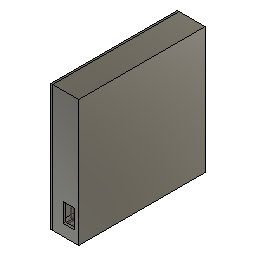
wifi-neopixel v1 (Autodesk Fusion 360 design; units mm, degrees)
Autodesk Fusion 360 part; units mm, degrees
(part 1 of 2)
sketch "Schizzo1" plane through (0, 0, 0) normal (1, 0, 0) x (0, 1, 0) in component "elettronica"
  line L0 (0, 0) -> (80, 0)
  line L1 (80, 0) -> (80, 80)
  line L2 (80, 80) -> (0, 80)
  line L3 (0, 80) -> (0, 0)
  line L4 (2, 77.5) -> (7, 77.5)
  line L5 (7, 77.5) -> (7, 72.5)
  line L6 (7, 72.5) -> (2, 72.5)
  line L7 (2, 72.5) -> (2, 77.5)
  line L8 (17, 72.5) -> (12, 72.5)
  line L9 (17, 77.5) -> (17, 72.5)
  line L10 (12, 77.5) -> (17, 77.5)
  line L11 (12, 72.5) -> (12, 77.5)
  line L12 (27, 72.5) -> (22, 72.5)
  line L13 (27, 77.5) -> (27, 72.5)
  line L14 (22, 77.5) -> (27, 77.5)
  line L15 (22, 72.5) -> (22, 77.5)
  line L16 (37, 72.5) -> (32, 72.5)
  line L17 (37, 77.5) -> (37, 72.5)
  line L18 (32, 77.5) -> (37, 77.5)
  line L19 (32, 72.5) -> (32, 77.5)
  line L20 (47, 72.5) -> (42, 72.5)
  line L21 (47, 77.5) -> (47, 72.5)
  line L22 (42, 77.5) -> (47, 77.5)
  line L23 (42, 72.5) -> (42, 77.5)
  line L24 (57, 72.5) -> (52, 72.5)
  line L25 (57, 77.5) -> (57, 72.5)
  line L26 (52, 77.5) -> (57, 77.5)
  line L27 (52, 72.5) -> (52, 77.5)
  line L28 (67, 72.5) -> (62, 72.5)
  line L29 (67, 77.5) -> (67, 72.5)
  line L30 (62, 77.5) -> (67, 77.5)
  line L31 (62, 72.5) -> (62, 77.5)
  line L32 (77, 72.5) -> (72, 72.5)
  line L33 (77, 77.5) -> (77, 72.5)
  line L34 (72, 77.5) -> (77, 77.5)
  line L35 (72, 72.5) -> (72, 77.5)
  line L36 (7, 62.5) -> (2, 62.5)
  line L37 (7, 67.5) -> (7, 62.5)
  line L38 (2, 67.5) -> (7, 67.5)
  line L39 (2, 62.5) -> (2, 67.5)
  line L40 (17, 62.5) -> (12, 62.5)
  line L41 (17, 67.5) -> (17, 62.5)
  line L42 (12, 67.5) -> (17, 67.5)
  line L43 (12, 62.5) -> (12, 67.5)
  line L44 (27, 62.5) -> (22, 62.5)
  line L45 (27, 67.5) -> (27, 62.5)
  line L46 (22, 67.5) -> (27, 67.5)
  line L47 (22, 62.5) -> (22, 67.5)
  line L48 (37, 62.5) -> (32, 62.5)
  line L49 (37, 67.5) -> (37, 62.5)
  line L50 (32, 67.5) -> (37, 67.5)
  line L51 (32, 62.5) -> (32, 67.5)
  line L52 (47, 62.5) -> (42, 62.5)
  line L53 (47, 67.5) -> (47, 62.5)
  line L54 (42, 67.5) -> (47, 67.5)
  line L55 (42, 62.5) -> (42, 67.5)
  line L56 (57, 62.5) -> (52, 62.5)
  line L57 (57, 67.5) -> (57, 62.5)
  line L58 (52, 67.5) -> (57, 67.5)
  line L59 (52, 62.5) -> (52, 67.5)
  line L60 (67, 62.5) -> (62, 62.5)
  line L61 (67, 67.5) -> (67, 62.5)
  line L62 (62, 67.5) -> (67, 67.5)
  line L63 (62, 62.5) -> (62, 67.5)
  line L64 (77, 62.5) -> (72, 62.5)
  line L65 (77, 67.5) -> (77, 62.5)
  line L66 (72, 67.5) -> (77, 67.5)
  line L67 (72, 62.5) -> (72, 67.5)
  line L68 (7, 52.5) -> (2, 52.5)
  line L69 (7, 57.5) -> (7, 52.5)
  line L70 (2, 57.5) -> (7, 57.5)
  line L71 (2, 52.5) -> (2, 57.5)
  line L72 (17, 52.5) -> (12, 52.5)
  line L73 (17, 57.5) -> (17, 52.5)
  line L74 (12, 57.5) -> (17, 57.5)
  line L75 (12, 52.5) -> (12, 57.5)
  line L76 (27, 52.5) -> (22, 52.5)
  line L77 (27, 57.5) -> (27, 52.5)
  line L78 (22, 57.5) -> (27, 57.5)
  line L79 (22, 52.5) -> (22, 57.5)
  line L80 (37, 52.5) -> (32, 52.5)
  line L81 (37, 57.5) -> (37, 52.5)
  line L82 (32, 57.5) -> (37, 57.5)
  line L83 (32, 52.5) -> (32, 57.5)
  line L84 (47, 52.5) -> (42, 52.5)
  line L85 (47, 57.5) -> (47, 52.5)
  line L86 (42, 57.5) -> (47, 57.5)
  line L87 (42, 52.5) -> (42, 57.5)
  line L88 (57, 52.5) -> (52, 52.5)
  line L89 (57, 57.5) -> (57, 52.5)
  line L90 (52, 57.5) -> (57, 57.5)
  line L91 (52, 52.5) -> (52, 57.5)
  line L92 (67, 52.5) -> (62, 52.5)
  line L93 (67, 57.5) -> (67, 52.5)
  line L94 (62, 57.5) -> (67, 57.5)
  line L95 (62, 52.5) -> (62, 57.5)
  line L96 (77, 52.5) -> (72, 52.5)
  line L97 (77, 57.5) -> (77, 52.5)
  line L98 (72, 57.5) -> (77, 57.5)
  line L99 (72, 52.5) -> (72, 57.5)
  line L100 (7, 42.5) -> (2, 42.5)
  line L101 (7, 47.5) -> (7, 42.5)
  line L102 (2, 47.5) -> (7, 47.5)
  line L103 (2, 42.5) -> (2, 47.5)
  line L104 (17, 42.5) -> (12, 42.5)
  line L105 (17, 47.5) -> (17, 42.5)
  line L106 (12, 47.5) -> (17, 47.5)
  line L107 (12, 42.5) -> (12, 47.5)
  line L108 (27, 42.5) -> (22, 42.5)
  line L109 (27, 47.5) -> (27, 42.5)
  line L110 (22, 47.5) -> (27, 47.5)
  line L111 (22, 42.5) -> (22, 47.5)
  line L112 (37, 42.5) -> (32, 42.5)
  line L113 (37, 47.5) -> (37, 42.5)
  line L114 (32, 47.5) -> (37, 47.5)
  line L115 (32, 42.5) -> (32, 47.5)
  line L116 (47, 42.5) -> (42, 42.5)
  line L117 (47, 47.5) -> (47, 42.5)
  line L118 (42, 47.5) -> (47, 47.5)
  line L119 (42, 42.5) -> (42, 47.5)
  line L120 (57, 42.5) -> (52, 42.5)
  line L121 (57, 47.5) -> (57, 42.5)
  line L122 (52, 47.5) -> (57, 47.5)
  line L123 (52, 42.5) -> (52, 47.5)
  line L124 (67, 42.5) -> (62, 42.5)
  line L125 (67, 47.5) -> (67, 42.5)
  line L126 (62, 47.5) -> (67, 47.5)
  line L127 (62, 42.5) -> (62, 47.5)
  line L128 (77, 42.5) -> (72, 42.5)
  line L129 (77, 47.5) -> (77, 42.5)
  line L130 (72, 47.5) -> (77, 47.5)
  line L131 (72, 42.5) -> (72, 47.5)
  line L132 (7, 32.5) -> (2, 32.5)
  line L133 (7, 37.5) -> (7, 32.5)
  line L134 (2, 37.5) -> (7, 37.5)
  line L135 (2, 32.5) -> (2, 37.5)
  line L136 (17, 32.5) -> (12, 32.5)
  line L137 (17, 37.5) -> (17, 32.5)
  line L138 (12, 37.5) -> (17, 37.5)
  line L139 (12, 32.5) -> (12, 37.5)
  line L140 (27, 32.5) -> (22, 32.5)
  line L141 (27, 37.5) -> (27, 32.5)
  line L142 (22, 37.5) -> (27, 37.5)
  line L143 (22, 32.5) -> (22, 37.5)
  line L144 (37, 32.5) -> (32, 32.5)
  line L145 (37, 37.5) -> (37, 32.5)
  line L146 (32, 37.5) -> (37, 37.5)
  line L147 (32, 32.5) -> (32, 37.5)
  line L148 (47, 32.5) -> (42, 32.5)
  line L149 (47, 37.5) -> (47, 32.5)
  line L150 (42, 37.5) -> (47, 37.5)
  line L151 (42, 32.5) -> (42, 37.5)
  line L152 (57, 32.5) -> (52, 32.5)
  line L153 (57, 37.5) -> (57, 32.5)
  line L154 (52, 37.5) -> (57, 37.5)
  line L155 (52, 32.5) -> (52, 37.5)
  line L156 (67, 32.5) -> (62, 32.5)
  line L157 (67, 37.5) -> (67, 32.5)
  line L158 (62, 37.5) -> (67, 37.5)
  line L159 (62, 32.5) -> (62, 37.5)
  line L160 (77, 32.5) -> (72, 32.5)
  line L161 (77, 37.5) -> (77, 32.5)
  line L162 (72, 37.5) -> (77, 37.5)
  line L163 (72, 32.5) -> (72, 37.5)
  line L164 (7, 22.5) -> (2, 22.5)
  line L165 (7, 27.5) -> (7, 22.5)
  line L166 (2, 27.5) -> (7, 27.5)
  line L167 (2, 22.5) -> (2, 27.5)
  line L168 (17, 22.5) -> (12, 22.5)
  line L169 (17, 27.5) -> (17, 22.5)
  line L170 (12, 27.5) -> (17, 27.5)
  line L171 (12, 22.5) -> (12, 27.5)
  line L172 (27, 22.5) -> (22, 22.5)
  line L173 (27, 27.5) -> (27, 22.5)
  line L174 (22, 27.5) -> (27, 27.5)
  line L175 (22, 22.5) -> (22, 27.5)
  line L176 (37, 22.5) -> (32, 22.5)
  line L177 (37, 27.5) -> (37, 22.5)
  line L178 (32, 27.5) -> (37, 27.5)
  line L179 (32, 22.5) -> (32, 27.5)
  line L180 (47, 22.5) -> (42, 22.5)
  line L181 (47, 27.5) -> (47, 22.5)
  line L182 (42, 27.5) -> (47, 27.5)
  line L183 (42, 22.5) -> (42, 27.5)
  line L184 (57, 22.5) -> (52, 22.5)
  line L185 (57, 27.5) -> (57, 22.5)
  line L186 (52, 27.5) -> (57, 27.5)
  line L187 (52, 22.5) -> (52, 27.5)
  line L188 (67, 22.5) -> (62, 22.5)
  line L189 (67, 27.5) -> (67, 22.5)
  line L190 (62, 27.5) -> (67, 27.5)
  line L191 (62, 22.5) -> (62, 27.5)
  line L192 (77, 22.5) -> (72, 22.5)
  line L193 (77, 27.5) -> (77, 22.5)
  line L194 (72, 27.5) -> (77, 27.5)
  line L195 (72, 22.5) -> (72, 27.5)
  line L196 (7, 12.5) -> (2, 12.5)
  line L197 (7, 17.5) -> (7, 12.5)
  line L198 (2, 17.5) -> (7, 17.5)
  line L199 (2, 12.5) -> (2, 17.5)
  line L200 (17, 12.5) -> (12, 12.5)
  line L201 (17, 17.5) -> (17, 12.5)
  line L202 (12, 17.5) -> (17, 17.5)
  line L203 (12, 12.5) -> (12, 17.5)
  line L204 (27, 12.5) -> (22, 12.5)
  line L205 (27, 17.5) -> (27, 12.5)
  line L206 (22, 17.5) -> (27, 17.5)
  line L207 (22, 12.5) -> (22, 17.5)
  line L208 (37, 12.5) -> (32, 12.5)
  line L209 (37, 17.5) -> (37, 12.5)
  line L210 (32, 17.5) -> (37, 17.5)
  line L211 (32, 12.5) -> (32, 17.5)
  line L212 (47, 12.5) -> (42, 12.5)
  line L213 (47, 17.5) -> (47, 12.5)
  line L214 (42, 17.5) -> (47, 17.5)
  line L215 (42, 12.5) -> (42, 17.5)
  line L216 (57, 12.5) -> (52, 12.5)
  line L217 (57, 17.5) -> (57, 12.5)
  line L218 (52, 17.5) -> (57, 17.5)
  line L219 (52, 12.5) -> (52, 17.5)
  line L220 (67, 12.5) -> (62, 12.5)
  line L221 (67, 17.5) -> (67, 12.5)
  line L222 (62, 17.5) -> (67, 17.5)
  line L223 (62, 12.5) -> (62, 17.5)
  line L224 (77, 12.5) -> (72, 12.5)
  line L225 (77, 17.5) -> (77, 12.5)
  line L226 (72, 17.5) -> (77, 17.5)
  line L227 (72, 12.5) -> (72, 17.5)
  line L228 (7, 2.5) -> (2, 2.5)
  line L229 (7, 7.5) -> (7, 2.5)
  line L230 (2, 7.5) -> (7, 7.5)
  line L231 (2, 2.5) -> (2, 7.5)
  line L232 (17, 2.5) -> (12, 2.5)
  line L233 (17, 7.5) -> (17, 2.5)
  line L234 (12, 7.5) -> (17, 7.5)
  line L235 (12, 2.5) -> (12, 7.5)
  line L236 (27, 2.5) -> (22, 2.5)
  line L237 (27, 7.5) -> (27, 2.5)
  line L238 (22, 7.5) -> (27, 7.5)
  line L239 (22, 2.5) -> (22, 7.5)
  line L240 (37, 2.5) -> (32, 2.5)
  line L241 (37, 7.5) -> (37, 2.5)
  line L242 (32, 7.5) -> (37, 7.5)
  line L243 (32, 2.5) -> (32, 7.5)
  line L244 (47, 2.5) -> (42, 2.5)
  line L245 (47, 7.5) -> (47, 2.5)
  line L246 (42, 7.5) -> (47, 7.5)
  line L247 (42, 2.5) -> (42, 7.5)
  line L248 (57, 2.5) -> (52, 2.5)
  line L249 (57, 7.5) -> (57, 2.5)
  line L250 (52, 7.5) -> (57, 7.5)
  line L251 (52, 2.5) -> (52, 7.5)
  line L252 (67, 2.5) -> (62, 2.5)
  line L253 (67, 7.5) -> (67, 2.5)
  line L254 (62, 7.5) -> (67, 7.5)
  line L255 (62, 2.5) -> (62, 7.5)
  line L256 (77, 2.5) -> (72, 2.5)
  line L257 (77, 7.5) -> (77, 2.5)
  line L258 (72, 7.5) -> (77, 7.5)
  line L259 (72, 2.5) -> (72, 7.5)
  dimension "d1" = 80
  dimension "d2" = 80
  dimension "d3" = 5
  dimension "d4" = 5
  dimension "d5" = 2
  dimension "d6" = 2.5
  dimension "d9" = 10
  dimension "d10" = -10
  constraint horizontal L0
  constraint vertical L1
  constraint horizontal L2
  constraint vertical L3
  constraint coincident L0.start L3.end
  constraint horizontal L4
  constraint vertical L5
  constraint horizontal L6
  constraint vertical L7
  measures "d1" distance of L0.start L0.end
  measures "d2" distance of L0.start L2.end
  measures "d3" distance of L4.start L4.end
  measures "d4" distance of L4.start L6.end
  measures "d5" distance of L3 L7
  measures "d6" distance of L2 L4
extrude "Estrusione1" add sketch "Schizzo1" against normal blind 0.4 contours L0 L1 L2 L3 | L4 L5 L6 L7 | L8 L9 L10 L11 | L12 L13 L14 L15 | L16 L17 L18 L19 | L20 L21 L22 L23 | L24 L25 L26 L27 | L28 L29 L30 L31 | L32 L33 L34 L35 | L36 L37 L38 L39 | L40 L41 L42 L43 | L44 L45 L46 L47 | L48 L49 L50 L51 | L52 L53 L54 L55 | L56 L57 L58 L59 | L60 L61 L62 L63 | L64 L65 L66 L67 | L68 L69 L70 L71 | L72 L73 L74 L75 | L76 L77 L78 L79 | L80 L81 L82 L83 | L84 L85 L86 L87 | L88 L89 L90 L91 | L92 L93 L94 L95 | L96 L97 L98 L99 | L100 L101 L102 L103 | L104 L105 L106 L107 | L108 L109 L110 L111 | L112 L113 L114 L115 | L116 L117 L118 L119 | L120 L121 L122 L123 | L124 L125 L126 L127 | L128 L129 L130 L131 | L132 L133 L134 L135 | L136 L137 L138 L139 | L140 L141 L142 L143 | L144 L145 L146 L147 | L148 L149 L150 L151 | L152 L153 L154 L155 | L156 L157 L158 L159 | L160 L161 L162 L163 | L164 L165 L166 L167 | L168 L169 L170 L171 | L172 L173 L174 L175 | L176 L177 L178 L179 | L180 L181 L182 L183 | L184 L185 L186 L187 | L188 L189 L190 L191 | L192 L193 L194 L195 | L196 L197 L198 L199 | L200 L201 L202 L203 | L204 L205 L206 L207 | L208 L209 L210 L211 | L212 L213 L214 L215 | L216 L217 L218 L219 | L220 L221 L222 L223 | L224 L225 L226 L227 | L228 L229 L230 L231 | L232 L233 L234 L235 | L236 L237 L238 L239 | L240 L241 L242 L243 | L244 L245 L246 L247 | L248 L249 L250 L251 | L252 L253 L254 L255 | L256 L257 L258 L259 makes body 1 in component "elettronica"
extrude "Estrusione2" add sketch "Schizzo1" along normal blind 1.4 contours L4 L5 L6 L7 | L8 L9 L10 L11 | L12 L13 L14 L15 | L16 L17 L18 L19 | L20 L21 L22 L23 | L24 L25 L26 L27 | L28 L29 L30 L31 | L32 L33 L34 L35 | L36 L37 L38 L39 | L40 L41 L42 L43 | L44 L45 L46 L47 | L48 L49 L50 L51 | L52 L53 L54 L55 | L56 L57 L58 L59 | L60 L61 L62 L63 | L64 L65 L66 L67 | L68 L69 L70 L71 | L72 L73 L74 L75 | L76 L77 L78 L79 | L80 L81 L82 L83 | L84 L85 L86 L87 | L88 L89 L90 L91 | L92 L93 L94 L95 | L96 L97 L98 L99 | L100 L101 L102 L103 | L104 L105 L106 L107 | L108 L109 L110 L111 | L112 L113 L114 L115 | L116 L117 L118 L119 | L120 L121 L122 L123 | L124 L125 L126 L127 | L128 L129 L130 L131 | L132 L133 L134 L135 | L136 L137 L138 L139 | L140 L141 L142 L143 | L144 L145 L146 L147 | L148 L149 L150 L151 | L152 L153 L154 L155 | L156 L157 L158 L159 | L160 L161 L162 L163 | L164 L165 L166 L167 | L168 L169 L170 L171 | L172 L173 L174 L175 | L176 L177 L178 L179 | L180 L181 L182 L183 | L184 L185 L186 L187 | L188 L189 L190 L191 | L192 L193 L194 L195 | L196 L197 L198 L199 | L200 L201 L202 L203 | L204 L205 L206 L207 | L208 L209 L210 L211 | L212 L213 L214 L215 | L216 L217 L218 L219 | L220 L221 L222 L223 | L224 L225 L226 L227 | L228 L229 L230 L231 | L232 L233 L234 L235 | L236 L237 L238 L239 | L240 L241 L242 L243 | L244 L245 L246 L247 | L248 L249 L250 L251 | L252 L253 L254 L255 | L256 L257 L258 L259 bodies 1 in component "elettronica"
sketch "Schizzo2" plane through (-0.4, 0, 0) normal (-1, 0, 0) x (0, -1, 0) in component "elettronica"
  line L0 (0, 0) -> (0, 80)
  line L1 (0, 80) -> (-80, 80)
  line L2 (-80, 80) -> (-80, 0)
  line L3 (-80, 0) -> (0, 0)
  line L4 (-61.5, 66) -> (-57.5, 66)
  line L5 (-57.5, 66) -> (-57.5, 64)
  line L6 (-57.5, 64) -> (-61.5, 64)
  line L7 (-61.5, 64) -> (-61.5, 66)
  line L8 (-61.5, 61) -> (-57.5, 61)
  line L9 (-57.5, 61) -> (-57.5, 59)
  line L10 (-57.5, 59) -> (-61.5, 59)
  line L11 (-61.5, 59) -> (-61.5, 61)
  line L12 (-61.5, 56) -> (-57.5, 56)
  line L13 (-57.5, 56) -> (-57.5, 54)
  line L14 (-57.5, 54) -> (-61.5, 54)
  line L15 (-61.5, 54) -> (-61.5, 56)
  line L16 (-61.5, 46) -> (-57.5, 46)
  line L17 (-57.5, 46) -> (-57.5, 44)
  line L18 (-57.5, 44) -> (-61.5, 44)
  line L19 (-61.5, 44) -> (-61.5, 46)
  line L20 (-61.5, 41) -> (-57.5, 41)
  line L21 (-57.5, 41) -> (-57.5, 39)
  line L22 (-57.5, 39) -> (-61.5, 39)
  line L23 (-61.5, 39) -> (-61.5, 41)
  line L24 (-61.5, 26) -> (-57.5, 26)
  line L25 (-57.5, 26) -> (-57.5, 24)
  line L26 (-57.5, 24) -> (-61.5, 24)
  line L27 (-61.5, 24) -> (-61.5, 26)
  line L28 (-61.5, 21) -> (-57.5, 21)
  line L29 (-57.5, 21) -> (-57.5, 19)
  line L30 (-57.5, 19) -> (-61.5, 19)
  line L31 (-61.5, 19) -> (-61.5, 21)
  line L32 (-61.5, 16) -> (-57.5, 16)
  line L33 (-57.5, 16) -> (-57.5, 14)
  line L34 (-57.5, 14) -> (-61.5, 14)
  line L35 (-61.5, 14) -> (-61.5, 16)
  dimension "d15" = 4
  dimension "d16" = 2
  dimension "d17" = 4
  dimension "d18" = 2
  dimension "d19" = 4
  dimension "d20" = 2
  dimension "d21" = 4
  dimension "d22" = 2
  dimension "d23" = 4
  dimension "d24" = 2
  dimension "d25" = 4
  dimension "d26" = 2
  dimension "d27" = 4
  dimension "d28" = 2
  dimension "d29" = 4
  dimension "d30" = 2
  dimension "d31" = 14
  dimension "d32" = 18.5
  dimension "d33" = 3
  dimension "d34" = 3
  dimension "d35" = 3
  dimension "d36" = 3
  dimension "d37" = 3
  dimension "d38" = 8
  dimension "d39" = 13
  constraint horizontal L4
  constraint vertical L5
  constraint horizontal L6
  constraint vertical L7
  constraint horizontal L8
  constraint vertical L9
  constraint horizontal L10
  constraint vertical L11
  constraint horizontal L12
  constraint vertical L13
  constraint horizontal L14
  constraint vertical L15
  constraint horizontal L16
  constraint vertical L17
  constraint horizontal L18
  constraint vertical L19
  constraint horizontal L20
  constraint vertical L21
  constraint horizontal L22
  constraint vertical L23
  constraint horizontal L24
  constraint vertical L25
  constraint horizontal L26
  constraint vertical L27
  constraint horizontal L28
  constraint vertical L29
  constraint horizontal L30
  constraint vertical L31
  constraint horizontal L32
  constraint vertical L33
  constraint horizontal L34
  constraint vertical L35
  constraint collinear L7 L11
  constraint collinear L11 L15
  constraint collinear L15 L19
  constraint collinear L19 L23
  constraint collinear L23 L27
  constraint collinear L27 L31
  constraint collinear L31 L35
  measures "d15" distance of L4.start L4.end
  measures "d16" distance of L4.start L6.end
  measures "d17" distance of L8.start L8.end
  measures "d18" distance of L8.start L10.end
  measures "d19" distance of L12.start L12.end
  measures "d20" distance of L12.start L14.end
  measures "d21" distance of L16.start L16.end
  measures "d22" distance of L16.start L18.end
  measures "d23" distance of L20.start L20.end
  measures "d24" distance of L20.start L22.end
  measures "d25" distance of L24.start L24.end
  measures "d26" distance of L24.start L26.end
  measures "d27" distance of L28.start L28.end
  measures "d28" distance of L28.start L30.end
  measures "d29" distance of L32.start L32.end
  measures "d30" distance of L32.start L34.end
  measures "d31" distance of L1 L4
  measures "d32" distance of L2 L7
  measures "d33" distance of L6 L8
  measures "d34" distance of L10 L12
  measures "d35" distance of L18 L20
  measures "d36" distance of L26 L28
  measures "d37" distance of L30 L32
  measures "d38" distance of L14 L16
  measures "d39" distance of L22 L24
extrude "Estrusione3" add sketch "Schizzo2" along normal blind 0.1 contours L4 L5 L6 L7 | L8 L9 L10 L11 | L12 L13 L14 L15 | L16 L17 L18 L19 | L20 L21 L22 L23 | L24 L25 L26 L27 | L28 L29 L30 L31 | L32 L33 L34 L35 bodies 1 in component "elettronica"
sketch "Schizzo3" plane through (0, 0, 0) normal (0, 0, 1) x (1, 0, 0) in component "elettronica"
  line L0 (22.5, -3.7) -> (54.5, -3.7)
  line L1 (54.5, -3.7) -> (54.5, 5)
  line L2 (54.5, 5) -> (53.9, 5)
  line L3 (53.3, 5.6) -> (53.3, 13.4)
  line L4 (53.9, 14) -> (54.5, 14)
  line L5 (54.5, 14) -> (54.5, 19.8)
  line L6 (54.5, 19.8) -> (49, 19.8)
  line L7 (47.1, 21.7) -> (47.1, 21.8)
  line L8 (47.1, 21.8) -> (22.5, 21.8)
  line L9 (20, 19.3) -> (20, -1.2)
  arc A0 (53.3, 5.6) -> (53.9, 5) centre (53.9, 5.6) ccw
  arc A1 (53.9, 14) -> (53.3, 13.4) centre (53.9, 13.4) ccw
  arc A2 (47.1, 21.7) -> (49, 19.8) centre (49, 21.7) ccw
  line L10 (22.5, 21.8) -> (20, 19.3)
  line L11 (22.5, -3.7) -> (20, -1.2)
  point P0 (20, -3.7)
  point P1 (53.3, 5)
  point P2 (53.3, 14)
  point P3 (47.1, 19.8)
  point P4 (20, 21.8)
  dimension "d42" = 34.5
  dimension "d43" = 1.2
  dimension "d44" = 9
  dimension "d45" = 25.5
  dimension "d46" = 2
  dimension "d47" = 8.7
  dimension "d48" = 7.4
  dimension "d49" = 0.6
  dimension "d50" = 1.9
  dimension "d51" = 2.5
  dimension "d52" = 2.5
  dimension "d53" = 2.5
  dimension "d54" = 2.5
  constraint horizontal L0
  constraint perpendicular L0 L1
  constraint perpendicular L1 L2
  constraint perpendicular L2 L3
  constraint perpendicular L1 L4
  constraint perpendicular L4 L5
  constraint perpendicular L5 L6
  constraint perpendicular L6 L7
  constraint perpendicular L7 L8
  constraint perpendicular L0 L9
  constraint collinear L1 L5
  constraint coincident P1 L2
  constraint coincident P1 L3
  constraint tangent L2 A0
  constraint tangent L3 A0
  constraint coincident P2 L3
  constraint coincident P2 L4
  constraint tangent L3 A1
  constraint tangent L4 A1
  constraint equal A0 A1
  constraint coincident P3 L6
  constraint coincident P3 L7
  constraint tangent L6 A2
  constraint tangent L7 A2
  constraint coincident P4 L8
  constraint coincident P4 L9
  constraint coincident P0 L0
  constraint coincident P0 L9
  measures "d42" distance of P0 L0.end
  measures "d43" distance of L1.end P1
  measures "d44" distance of P1 P2
  measures "d45" distance of P0 P4
  measures "d46" distance of P3 L7.end
  measures "d47" distance of L0.end L1.end
  measures "d48" distance of L5.end P3
  measures "d49" radius of A0
  measures "d50" radius of A2
  measures "d51" distance of P4 L8.end
  measures "d52" distance of P4 L9.start
  measures "d53" distance of P0 L0.start
  measures "d54" distance of P0 L9.end
extrude "Estrusione4" add sketch "Schizzo3" along normal blind 1 separate body makes body 2 in component "elettronica"
sketch "Schizzo4" plane through (0, 0, 1) normal (0, 0, 1) x (-1, 0, 0) in component "elettronica"
  line L0 (-54.5, 3.7) -> (-54.5, -5)
  line L1 (-54.5, -5) -> (-53.9, -5)
  arc A0 (-53.3, -5.6) -> (-53.9, -5) centre (-53.9, -5.6) ccw
  line L2 (-53.3, -5.6) -> (-53.3, -13.4)
  arc A1 (-53.9, -14) -> (-53.3, -13.4) centre (-53.9, -13.4) ccw
  line L3 (-53.9, -14) -> (-54.5, -14)
  line L4 (-54.5, -14) -> (-54.5, -19.8)
  line L5 (-54.5, -19.8) -> (-49, -19.8)
  arc A2 (-47.1, -21.7) -> (-49, -19.8) centre (-49, -21.7) ccw
  line L6 (-47.1, -21.7) -> (-47.1, -21.8)
  line L7 (-47.1, -21.8) -> (-22.5, -21.8)
  line L8 (-22.5, -21.8) -> (-20, -19.3)
  line L9 (-20, -19.3) -> (-20, 1.2)
  line L10 (-20, 1.2) -> (-22.5, 3.7)
  line L11 (-22.5, 3.7) -> (-54.5, 3.7)
  line L12 (-48.6, -19.8) -> (-53, -19.8)
  line L13 (-53, -19.8) -> (-53, -17.4)
  line L14 (-53, -17.4) -> (-48.6, -17.4)
  line L15 (-48.6, -17.4) -> (-48.6, -19.8)
  dimension "d57" = 4.4
  dimension "d58" = 2.4
  dimension "d59" = 1.5
  constraint horizontal L12
  constraint vertical L13
  constraint horizontal L14
  constraint vertical L15
  constraint coincident L5 L12.start
  measures "d57" distance of L12.start L12.end
  measures "d58" distance of L12.start L14.end
  measures "d59" distance of L4 L13
extrude "Estrusione5" add sketch "Schizzo4" along normal blind 2 contours L5 L12 L13 L14 L15 bodies 2 in component "elettronica"
sketch "Schizzo5" plane through (0, 19.8, 0) normal (0, 1, 0) x (-1, 0, 0) in component "elettronica"
  line L0 (-54.5, 0) -> (-49, 0)
  line L1 (-49, 0) -> (-49, 1)
  line L2 (-49, 1) -> (-48.6, 1)
  line L3 (-48.6, 1) -> (-48.6, 3)
  line L4 (-48.6, 3) -> (-53, 3)
  line L5 (-53, 3) -> (-53, 1)
  line L6 (-53, 1) -> (-54.5, 1)
  line L7 (-54.5, 1) -> (-54.5, 0)
  line L8 (-48.6, 3) -> (-53, 1) construction
  line L9 (-53, 3) -> (-48.6, 1) construction
  line L10 (-49.8, 2.5) -> (-51.8, 2.5)
  line L11 (-51.8, 2.5) -> (-51.8, 1.5)
  line L12 (-51.8, 1.5) -> (-49.8, 1.5)
  line L13 (-49.8, 1.5) -> (-49.8, 2.5)
  line L14 (-49.8, 2.5) -> (-51.8, 1.5) construction
  line L15 (-51.8, 2.5) -> (-49.8, 1.5) construction
  point P0 (-50.8, 2)
  dimension "d62" = 2
  dimension "d63" = 1
  constraint coincident L3.end L4.start
  constraint coincident L5.end L6.start
  constraint coincident L4.end L5.start
  constraint coincident L2.end L3.start
  constraint horizontal L10
  constraint perpendicular L10 L11
  constraint parallel L10 L12
  constraint parallel L11 L13
  constraint coincident L14 P0
  constraint coincident L15 P0
  constraint midpoint L9 P0
  measures "d62" distance of L11.end L12.end
  measures "d63" distance of L10.end L11.end
extrude "Estrusione6" add sketch "Schizzo5" along normal blind 1 contours L10 L11 L12 L13 bodies 2 in component "elettronica"
sketch "Schizzo6" plane through (0, 0, 1) normal (0, 0, 1) x (-1, 0, 0) in component "elettronica"
  line L0 (-53, -19.8) -> (-53, -17.4)
  line L1 (-53, -17.4) -> (-48.6, -17.4)
  line L2 (-48.6, -17.4) -> (-48.6, -19.8)
  line L3 (-48.6, -19.8) -> (-49, -19.8)
  arc A0 (-47.1, -21.7) -> (-49, -19.8) centre (-49, -21.7) ccw
  line L4 (-47.1, -21.7) -> (-47.1, -21.8)
  line L5 (-47.1, -21.8) -> (-22.5, -21.8)
  line L6 (-22.5, -21.8) -> (-20, -19.3)
  line L7 (-20, -19.3) -> (-20, 1.2)
  line L8 (-20, 1.2) -> (-22.5, 3.7)
  line L9 (-22.5, 3.7) -> (-54.5, 3.7)
  line L10 (-54.5, 3.7) -> (-54.5, -5)
  line L11 (-54.5, -5) -> (-53.9, -5)
  arc A1 (-53.3, -5.6) -> (-53.9, -5) centre (-53.9, -5.6) ccw
  line L12 (-53.3, -5.6) -> (-53.3, -13.4)
  arc A2 (-53.9, -14) -> (-53.3, -13.4) centre (-53.9, -13.4) ccw
  line L13 (-53.9, -14) -> (-54.5, -14)
  line L14 (-54.5, -14) -> (-54.5, -19.8)
  line L15 (-54.5, -19.8) -> (-53, -19.8)
  line L16 (-40.1, -15.3) -> (-44.1, -15.3)
  line L17 (-44.1, -15.3) -> (-44.1, -5.3)
  line L18 (-44.1, -5.3) -> (-40.1, -5.3)
  line L19 (-40.1, -5.3) -> (-40.1, -15.3)
  dimension "d66" = 4
  dimension "d67" = 10
  dimension "d68" = 10.4
  dimension "d69" = 6.5
  constraint horizontal L16
  constraint vertical L17
  constraint horizontal L18
  constraint vertical L19
  measures "d66" distance of L16.start L16.end
  measures "d67" distance of L16.start L18.end
  measures "d68" distance of L14 L17
  measures "d69" distance of L5 L16
extrude "Estrusione7" add sketch "Schizzo6" along normal blind 2 contours L16 L17 L18 L19 bodies 2 in component "elettronica"
sketch "Schizzo7" plane through (0, 0, 1) normal (0, 0, 1) x (-1, 0, 0) in component "elettronica"
  line L0 (-40.1, -5.3) -> (-40.1, -15.3)
  line L1 (-40.1, -15.3) -> (-44.1, -15.3)
  line L2 (-44.1, -15.3) -> (-44.1, -5.3)
  line L3 (-44.1, -5.3) -> (-40.1, -5.3)
  line L4 (-53, -19.8) -> (-53, -17.4)
  line L5 (-53, -17.4) -> (-48.6, -17.4)
  line L6 (-48.6, -17.4) -> (-48.6, -19.8)
  line L7 (-48.6, -19.8) -> (-49, -19.8)
  arc A0 (-47.1, -21.7) -> (-49, -19.8) centre (-49, -21.7) ccw
  line L8 (-47.1, -21.7) -> (-47.1, -21.8)
  line L9 (-47.1, -21.8) -> (-22.5, -21.8)
  line L10 (-22.5, -21.8) -> (-20, -19.3)
  line L11 (-20, -19.3) -> (-20, 1.2)
  line L12 (-20, 1.2) -> (-22.5, 3.7)
  line L13 (-22.5, 3.7) -> (-54.5, 3.7)
  line L14 (-54.5, 3.7) -> (-54.5, -5)
  line L15 (-54.5, -5) -> (-53.9, -5)
  arc A1 (-53.3, -5.6) -> (-53.9, -5) centre (-53.9, -5.6) ccw
  line L16 (-53.3, -5.6) -> (-53.3, -13.4)
  arc A2 (-53.9, -14) -> (-53.3, -13.4) centre (-53.9, -13.4) ccw
  line L17 (-53.9, -14) -> (-54.5, -14)
  line L18 (-54.5, -14) -> (-54.5, -19.8)
  line L19 (-54.5, -19.8) -> (-53, -19.8)
  line L20 (-48.3, -13.6) -> (-53.9, -13.6)
  line L21 (-53.9, -13.6) -> (-53.9, -6.1)
  line L22 (-53.9, -6.1) -> (-48.3, -6.1)
  line L23 (-48.3, -6.1) -> (-48.3, -13.6)
  dimension "d72" = 5.6
  dimension "d73" = 7.5
  dimension "d74" = 4.2
  dimension "d75" = 3.8
  constraint horizontal L20
  constraint vertical L21
  constraint horizontal L22
  constraint vertical L23
  measures "d72" distance of L20.start L20.end
  measures "d73" distance of L20.start L22.end
  measures "d74" distance of L2 L23
  measures "d75" distance of L5 L20
extrude "Estrusione8" add sketch "Schizzo7" along normal blind 2.2 contours L16 A2 L20 L21 L22 | L16 A2 L20 L22 L23 bodies 2 in component "elettronica"
chamfer "Smusso1" distance 1.05 angle 45 2 edges at (53.6, 6.1, 1) (53.6172, 13.6, 1) on bodies 2 in component "elettronica"
fillet "Raccordo1" radius 0.25 2 edges at (51.1, 6.1, 3.2) (51.1, 13.6, 3.2) on bodies 2 in component "elettronica"
sketch "Schizzo8" plane through (53.9, 0, 0) normal (1, 0, 0) x (0, 1, 0) in component "elettronica"
  arc A0 (13.6, 2.95) -> (13.35, 3.2) centre (13.35, 2.95) ccw
  line L0 (13.35, 3.2) -> (6.35, 3.2)
  arc A1 (6.35, 3.2) -> (6.1, 2.95) centre (6.35, 2.95) ccw
  line L1 (6.1, 2.95) -> (6.1, 2.05)
  line L2 (6.1, 2.05) -> (7.15, 1)
  line L3 (7.15, 1) -> (12.55, 1)
  line L4 (12.55, 1) -> (13.6, 2.05)
  line L5 (13.6, 2.05) -> (13.6, 2.95)
  line L6 (6.3, 2.95) -> (6.3, 2.1328)
  line L7 (6.3, 2.1328) -> (7.2328, 1.2)
  line L8 (7.2328, 1.2) -> (12.4672, 1.2)
  line L9 (12.4672, 1.2) -> (13.4, 2.1328)
  line L10 (13.4, 2.1328) -> (13.4, 2.95)
  arc A2 (13.4, 2.95) -> (13.35, 3) centre (13.35, 2.95) ccw
  line L11 (13.35, 3) -> (6.35, 3)
  arc A3 (6.35, 3) -> (6.3, 2.95) centre (6.35, 2.95) ccw
  dimension "d81" = -0.2
extrude "Estrusione9" cut sketch "Schizzo8" against normal blind 3 contours L6 L7 L8 L9 L10 A2 L11 A3 bodies 2 in component "elettronica"
sketch "Schizzo9" plane through (0, 0, 1) normal (0, 0, 1) x (-1, 0, 0) in component "elettronica"
  line L0 (-48.3, -13.6) -> (-53.3343, -13.6)
  arc A0 (-53.9, -14) -> (-53.3343, -13.6) centre (-53.9, -13.4) ccw
  line L1 (-53.9, -14) -> (-54.5, -14)
  line L2 (-54.5, -14) -> (-54.5, -19.8)
  line L3 (-54.5, -19.8) -> (-53, -19.8)
  line L4 (-53, -19.8) -> (-53, -17.4)
  line L5 (-53, -17.4) -> (-48.6, -17.4)
  line L6 (-48.6, -17.4) -> (-48.6, -19.8)
  line L7 (-48.6, -19.8) -> (-49, -19.8)
  arc A1 (-47.1, -21.7) -> (-49, -19.8) centre (-49, -21.7) ccw
  line L8 (-47.1, -21.7) -> (-47.1, -21.8)
  line L9 (-47.1, -21.8) -> (-22.5, -21.8)
  line L10 (-22.5, -21.8) -> (-20, -19.3)
  line L11 (-20, -19.3) -> (-20, 1.2)
  line L12 (-20, 1.2) -> (-22.5, 3.7)
  line L13 (-22.5, 3.7) -> (-54.5, 3.7)
  line L14 (-54.5, 3.7) -> (-54.5, -5)
  line L15 (-54.5, -5) -> (-53.9, -5)
  arc A2 (-53.3, -5.6) -> (-53.9, -5) centre (-53.9, -5.6) ccw
  line L16 (-53.3, -5.6) -> (-53.3, -6.1)
  line L17 (-53.3, -6.1) -> (-48.3, -6.1)
  line L18 (-48.3, -6.1) -> (-48.3, -13.6)
  line L19 (-40.1, -5.3) -> (-40.1, -15.3)
  line L20 (-40.1, -15.3) -> (-44.1, -15.3)
  line L21 (-44.1, -15.3) -> (-44.1, -5.3)
  line L22 (-44.1, -5.3) -> (-40.1, -5.3)
  circle A3 centre (-27, -20.6) radius 0.4
  circle A4 centre (-29.54, -20.6) radius 0.4
  circle A5 centre (-32.08, -20.6) radius 0.4
  circle A6 centre (-34.62, -20.6) radius 0.4
  circle A7 centre (-37.16, -20.6) radius 0.4
  circle A8 centre (-39.7, -20.6) radius 0.4
  circle A9 centre (-42.24, -20.6) radius 0.4
  circle A10 centre (-44.78, -20.6) radius 0.4
  circle A11 centre (-27, 2.5) radius 0.4
  circle A12 centre (-29.54, 2.5) radius 0.4
  circle A13 centre (-32.08, 2.5) radius 0.4
  circle A14 centre (-34.62, 2.5) radius 0.4
  circle A15 centre (-37.16, 2.5) radius 0.4
  circle A16 centre (-39.7, 2.5) radius 0.4
  circle A17 centre (-42.24, 2.5) radius 0.4
  circle A18 centre (-44.78, 2.5) radius 0.4
  dimension "d84" = 0.8
  dimension "d85" = 7
  dimension "d86" = 1.2
  dimension "d89" = -2.54
  dimension "d90" = 23.1
  measures "d84" diameter of A3
  measures "d85" distance of L11 A3.centre
  measures "d86" distance of L9 A3.centre
extrude "Estrusione10" cut sketch "Schizzo9" against normal through all contours A3 | A4 | A5 | A6 | A7 | A8 | A9 | A10 | A11 | A12 | A13 | A14 | A15 | A16 | A17 | A18 bodies 2 in component "elettronica"
sketch "Schizzo10" plane through (0, 0, 0) normal (0, 0, -1) x (1, 0, 0) in component "elettronica"
  circle A0 centre (39.7, 2.5) radius 0.4
  circle A1 centre (29.54, 2.5) radius 0.4
  circle A2 centre (39.7, -20.6) radius 0.4
  circle A3 centre (29.54, -20.6) radius 0.4
  circle A4 centre (32.08, -20.6) radius 0.4
  circle A5 centre (42.24, -20.6) radius 0.4
  circle A6 centre (32.08, 2.5) radius 0.4
  circle A7 centre (42.24, 2.5) radius 0.4
  circle A8 centre (37.16, 2.5) radius 0.4
  circle A9 centre (27, 2.5) radius 0.4
  circle A10 centre (37.16, -20.6) radius 0.4
  circle A11 centre (27, -20.6) radius 0.4
  circle A12 centre (34.62, -20.6) radius 0.4
  circle A13 centre (44.78, -20.6) radius 0.4
  circle A14 centre (34.62, 2.5) radius 0.4
  circle A15 centre (44.78, 2.5) radius 0.4
  line L0 (54.5, -5) -> (54.5, 3.7)
  line L1 (54.5, 3.7) -> (22.5, 3.7)
  line L2 (22.5, 3.7) -> (20, 1.2)
  line L3 (20, 1.2) -> (20, -19.3)
  line L4 (20, -19.3) -> (22.5, -21.8)
  line L5 (22.5, -21.8) -> (47.1, -21.8)
  line L6 (47.1, -21.8) -> (47.1, -21.7)
  arc A16 (49, -19.8) -> (47.1, -21.7) centre (49, -21.7) ccw
  line L7 (49, -19.8) -> (54.5, -19.8)
  line L8 (54.5, -19.8) -> (54.5, -14)
  line L9 (54.5, -14) -> (53.9, -14)
  arc A17 (53.3, -13.4) -> (53.9, -14) centre (53.9, -13.4) ccw
  line L10 (53.3, -13.4) -> (53.3, -5.6)
  arc A18 (53.9, -5) -> (53.3, -5.6) centre (53.9, -5.6) ccw
  line L11 (53.9, -5) -> (54.5, -5)
  line L12 (20, -1.3) -> (44, -1.3)
  line L13 (44, -1.3) -> (44, -17.3)
  line L14 (44, -17.3) -> (20, -17.3)
  line L15 (20, -17.3) -> (20, -1.3)
  dimension "d92" = 24
  dimension "d93" = 16
  dimension "d94" = 5
  constraint horizontal L12
  constraint vertical L13
  constraint horizontal L14
  constraint vertical L15
  constraint coincident L3 L12.start
  measures "d92" distance of L12.start L12.end
  measures "d93" distance of L12.start L14.end
  measures "d94" distance of L1 L12
extrude "Estrusione11" add sketch "Schizzo10" along normal blind 0.7 contours L3 L12 L13 L14 L15 bodies 2 in component "elettronica"
sketch "Schizzo11" plane through (0, 0, -0.7) normal (0, 0, -1) x (1, 0, 0) in component "elettronica"
  line L0 (20, -17.3) -> (44, -17.3)
  line L1 (44, -17.3) -> (44, -1.3)
  line L2 (44, -1.3) -> (20, -1.3)
  line L3 (20, -1.3) -> (20, -17.3)
  line L4 (27.8, -3.3) -> (42.8, -3.3)
  line L5 (42.8, -3.3) -> (42.8, -15.3)
  line L6 (42.8, -15.3) -> (27.8, -15.3)
  line L7 (27.8, -15.3) -> (27.8, -3.3)
  dimension "d97" = 15
  dimension "d98" = 12
  dimension "d99" = 1.2
  dimension "d100" = 2
  constraint horizontal L4
  constraint vertical L5
  constraint horizontal L6
  constraint vertical L7
  measures "d97" distance of L4.start L4.end
  measures "d98" distance of L4.start L6.end
  measures "d99" distance of L1 L5
  measures "d100" distance of L0 L6
extrude "Estrusione12" add sketch "Schizzo11" along normal blind 2.2 contours L4 L5 L6 L7 bodies 2 in component "elettronica"
sketch "Schizzo1 (2)" plane through (0, 0, 0) normal (1, 0, 0) x (0, 1, 0) in component "case"
  line L0 (80, 80) -> (80, 0)
  line L1 (0, 80) -> (80, 80)
  line L2 (80, 0) -> (0, 0)
  line L3 (0, 0) -> (0, 80)
  line L4 (-0.2, -0.2) -> (-0.2, 80.2)
  line L5 (-0.2, 80.2) -> (80.2, 80.2)
  line L6 (80.2, 80.2) -> (80.2, -0.2)
  line L7 (80.2, -0.2) -> (-0.2, -0.2)
  line L8 (-1.8, -1.8) -> (-1.8, 81.8)
  line L9 (-1.8, 81.8) -> (81.8, 81.8)
  line L10 (81.8, 81.8) -> (81.8, -1.8)
  line L11 (81.8, -1.8) -> (-1.8, -1.8)
  dimension "d103" = -0.2
  dimension "d104" = -1.8
extrude "Estrusione1'" add sketch "Schizzo1 (2)" along normal blind 1.2 separate body contours L0 L1 L2 L3 | L4 L5 L6 L7 | L8 L9 L10 L11 makes body 3 in component "case"
extrude "Estrusione2'" add sketch "Schizzo1 (2)" against normal blind 16 contours L8 L9 L10 L11 bodies 3 in component "case"
move_body "Sposta1" bodies 1 to x (1, 0, 0) y (0, 1, 0) z (0, 0, 1) at (-2.5162, 0, 0) in component "elettronica"
sketch "Schizzo2 (2)" plane through (-2.9162, 0, 0) normal (-1, 0, 0) x (0, -1, 0) in component "case"
  line L0 (-61.5, 14) -> (-61.5, 16)
  line L1 (-61.5, 16) -> (-57.5, 16)
  line L2 (-57.5, 16) -> (-57.5, 14)
  line L3 (-57.5, 14) -> (-61.5, 14)
  line L4 (-61.5, 44) -> (-61.5, 46)
  line L5 (-61.5, 46) -> (-57.5, 46)
  line L6 (-57.5, 46) -> (-57.5, 44)
  line L7 (-57.5, 44) -> (-61.5, 44)
  line L8 (-61.5, 64) -> (-61.5, 66)
  line L9 (-61.5, 66) -> (-57.5, 66)
  line L10 (-57.5, 66) -> (-57.5, 64)
  line L11 (-57.5, 64) -> (-61.5, 64)
  line L12 (-61.5, 39) -> (-61.5, 41)
  line L13 (-61.5, 41) -> (-57.5, 41)
  line L14 (-57.5, 41) -> (-57.5, 39)
  line L15 (-57.5, 39) -> (-61.5, 39)
  line L16 (-61.5, 19) -> (-61.5, 21)
  line L17 (-61.5, 21) -> (-57.5, 21)
  line L18 (-57.5, 21) -> (-57.5, 19)
  line L19 (-57.5, 19) -> (-61.5, 19)
  line L20 (-61.5, 54) -> (-61.5, 56)
  line L21 (-61.5, 56) -> (-57.5, 56)
  line L22 (-57.5, 56) -> (-57.5, 54)
  line L23 (-57.5, 54) -> (-61.5, 54)
  line L24 (-61.5, 59) -> (-61.5, 61)
  line L25 (-61.5, 61) -> (-57.5, 61)
  line L26 (-57.5, 61) -> (-57.5, 59)
  line L27 (-57.5, 59) -> (-61.5, 59)
  line L28 (-61.5, 24) -> (-61.5, 26)
  line L29 (-61.5, 26) -> (-57.5, 26)
  line L30 (-57.5, 26) -> (-57.5, 24)
  line L31 (-57.5, 24) -> (-61.5, 24)
  line L32 (0, 0) -> (0, 80)
  line L33 (0, 80) -> (-80, 80)
  line L34 (-80, 80) -> (-80, 0)
  line L35 (-80, 0) -> (0, 0)
  line L36 (-80.2, -0.2) -> (-80.2, 80.2)
  line L37 (-80.2, 80.2) -> (0.2, 80.2)
  line L38 (0.2, 80.2) -> (0.2, -0.2)
  line L39 (0.2, -0.2) -> (-80.2, -0.2)
  line L40 (-4.8, 75.2) -> (-4.8, 4.8)
  line L41 (-4.8, 4.8) -> (-75.2, 4.8)
  line L42 (-75.2, 4.8) -> (-75.2, 75.2)
  line L43 (-75.2, 75.2) -> (-4.8, 75.2)
  line L44 (-75.2, 75.2) -> (-4.8, 4.8) construction
  line L45 (-4.8, 75.2) -> (-75.2, 4.8) construction
  line L46 (-37.5, 75.2) -> (-42.5, 75.2)
  line L47 (-42.5, 75.2) -> (-42.5, 4.8)
  line L48 (-42.5, 4.8) -> (-37.5, 4.8)
  line L49 (-37.5, 4.8) -> (-37.5, 75.2)
  line L50 (-37.5, 75.2) -> (-42.5, 4.8) construction
  line L51 (-42.5, 75.2) -> (-37.5, 4.8) construction
  line L52 (-75.2, 52.3984) -> (-4.8, 52.3984)
  line L53 (-4.8, 52.3984) -> (-4.8, 47.3984)
  line L54 (-4.8, 47.3984) -> (-75.2, 47.3984)
  line L55 (-75.2, 47.3984) -> (-75.2, 52.3984)
  line L56 (-75.2, 32.5498) -> (-4.8, 32.5498)
  line L57 (-4.8, 32.5498) -> (-4.8, 27.5498)
  line L58 (-4.8, 27.5498) -> (-75.2, 27.5498)
  line L59 (-75.2, 27.5498) -> (-75.2, 32.5498)
  point P0 (-40, 40)
  dimension "d109" = 5
  dimension "d110" = 5
  dimension "d111" = 5
  dimension "d112" = 5
  constraint horizontal L46
  constraint perpendicular L46 L47
  constraint parallel L46 L48
  constraint parallel L47 L49
  constraint coincident L50 P0
  constraint coincident L51 P0
  constraint midpoint L45 P0
  constraint horizontal L52
  constraint vertical L53
  constraint horizontal L54
  constraint vertical L55
  constraint coincident L42 L52.start
  constraint horizontal L56
  constraint vertical L57
  constraint horizontal L58
  constraint vertical L59
  constraint coincident L42 L56.start
  measures "d110" distance of L47.end L48.end
  measures "d111" distance of L52.start L54.end
  measures "d112" distance of L56.start L58.end
extrude "Estrusione3'" add sketch "Schizzo2 (2)" along normal blind 1.2 separate body contours L32 L33 L34 L35 | L40 L49 L52 L53 L54 | L43 L46 L47 L49 L52 | L47 L49 L52 L54 | L40 L49 L56 L57 L58 | L47 L49 L54 L56 | L42 L47 L52 L54 L55 | L47 L49 L56 L58 | L41 L47 L48 L49 L58 | L42 L47 L56 L58 L59 makes body 4 in component "case"
move_body "Sposta2" bodies 2 to x (0, -1, 0) y (0, 0, -1) z (1, 0, 0) at (-12.4224, 55.8406, 22.4383) in component "elettronica"
move_body "Sposta3" bodies 2 to x (1, 0, 0) y (0, 1, 0) z (0, 0, 1) at (4.9521, -1.942, -0.6855) in component "elettronica"
move_body "Sposta4" bodies 2 to x (1, 0, 0) y (0, 1, 0) z (0, 0, 1) at (0, 0.6178, 0.0742) in component "elettronica"
sketch "Schizzo3 (2)" plane through (-4.1162, 0, 0) normal (-1, 0, 0) x (0, -1, 0) in component "case"
  line L0 (-75.2, 27.5498) -> (-42.5, 27.5498)
  line L1 (-42.5, 27.5498) -> (-42.5, 4.8)
  line L2 (-42.5, 4.8) -> (-75.2, 4.8)
  line L3 (-75.2, 4.8) -> (-75.2, 27.5498)
  line L4 (-75.2, 47.3984) -> (-42.5, 47.3984)
  line L5 (-42.5, 47.3984) -> (-42.5, 32.5498)
  line L6 (-42.5, 32.5498) -> (-75.2, 32.5498)
  line L7 (-75.2, 32.5498) -> (-75.2, 47.3984)
  line L8 (-75.2, 52.3984) -> (-75.2, 75.2)
  line L9 (-75.2, 75.2) -> (-42.5, 75.2)
  line L10 (-42.5, 75.2) -> (-42.5, 52.3984)
  line L11 (-42.5, 52.3984) -> (-75.2, 52.3984)
  line L12 (-4.8, 27.5498) -> (-4.8, 4.8)
  line L13 (-4.8, 4.8) -> (-37.5, 4.8)
  line L14 (-37.5, 4.8) -> (-37.5, 27.5498)
  line L15 (-37.5, 27.5498) -> (-4.8, 27.5498)
  line L16 (-4.8, 52.3984) -> (-37.5, 52.3984)
  line L17 (-37.5, 52.3984) -> (-37.5, 75.2)
  line L18 (-37.5, 75.2) -> (-4.8, 75.2)
  line L19 (-4.8, 75.2) -> (-4.8, 52.3984)
  line L20 (-37.5, 47.3984) -> (-4.8, 47.3984)
  line L21 (-4.8, 47.3984) -> (-4.8, 32.5498)
  line L22 (-4.8, 32.5498) -> (-37.5, 32.5498)
  line L23 (-37.5, 32.5498) -> (-37.5, 47.3984)
  line L24 (-80, 0) -> (0, 0)
  line L25 (0, 0) -> (0, 80)
  line L26 (0, 80) -> (-80, 80)
  line L27 (-80, 80) -> (-80, 0)
  line L28 (-32.0165, 25.5269) -> (-0.0165, 25.5269) construction
  line L29 (-32.0165, 25.5269) -> (-34.5165, 23.0269) construction
  line L30 (-34.5165, 20.5269) -> (-34.5165, 23.0269) construction
  line L31 (-34.5165, 20.5269) -> (-34.5165, 4.5269) construction
  line L32 (-34.5165, 2.5269) -> (-34.5165, 4.5269) construction
  line L33 (-32.0165, 0.0269) -> (-34.5165, 2.5269) construction
  line L34 (-7.4165, 0.0269) -> (-32.0165, 0.0269) construction
  line L35 (-4.8, 28.0269) -> (0, 28.0269)
  line L36 (0, 28.0269) -> (0, 23.0269)
  line L37 (0, 23.0269) -> (-4.8, 23.0269)
  line L38 (-4.8, 23.0269) -> (-4.8, 28.0269)
  line L39 (-32.0165, 27.5498) -> (-32.0165, 4.8)
  dimension "d115" = 5
  dimension "d116" = 2.5
  dimension "d117" = 2.5
  constraint horizontal L35
  constraint vertical L36
  constraint horizontal L37
  constraint vertical L38
  constraint coincident L12 L35.start
  constraint coincident L15 L39.start
  constraint coincident L13 L39.end
  constraint perpendicular L13 L39
  measures "d115" distance of L35.start L37.end
  measures "d116" distance of L28 L35
  measures "d117" distance of L31 L39
extrude "Estrusione4'" add sketch "Schizzo3 (2)" against normal up to surface (1.2 mm away) contours L13 L14 L15 L39 bodies 4 in component "case"
move_body "Sposta7" bodies 1 to x (1, 0, 0) y (0, 1, 0) z (0, 0, 1) at (0.8, 0, 0) in component "elettronica"
move_body "Sposta2'" bodies 4 to x (1, 0, 0) y (0, 1, 0) z (0, 0, 1) at (0.8, 0, 0) in component "case"
sketch "Schizzo10 (2)" plane through (-3.3162, 0, 0) normal (-1, 0, 0) x (0, -1, 0) in component "case"
  line L0 (-37.5, 47.3984) -> (-4.8, 47.3984)
  line L1 (-4.8, 47.3984) -> (-4.8, 32.5498)
  line L2 (-4.8, 32.5498) -> (-37.5, 32.5498)
  line L3 (-37.5, 32.5498) -> (-37.5, 47.3984)
  line L4 (-75.2, 27.5498) -> (-42.5, 27.5498)
  line L5 (-42.5, 27.5498) -> (-42.5, 4.8)
  line L6 (-42.5, 4.8) -> (-75.2, 4.8)
  line L7 (-75.2, 4.8) -> (-75.2, 27.5498)
  line L8 (-4.8, 27.5498) -> (-4.8, 4.8)
  line L9 (-4.8, 4.8) -> (-32.0165, 4.8)
  line L10 (-32.0165, 4.8) -> (-32.0165, 27.5498)
  line L11 (-32.0165, 27.5498) -> (-4.8, 27.5498)
  line L12 (-75.2, 47.3984) -> (-42.5, 47.3984)
  line L13 (-42.5, 47.3984) -> (-42.5, 32.5498)
  line L14 (-42.5, 32.5498) -> (-75.2, 32.5498)
  line L15 (-75.2, 32.5498) -> (-75.2, 47.3984)
  line L16 (-4.8, 52.3984) -> (-37.5, 52.3984)
  line L17 (-37.5, 52.3984) -> (-37.5, 75.2)
  line L18 (-37.5, 75.2) -> (-4.8, 75.2)
  line L19 (-4.8, 75.2) -> (-4.8, 52.3984)
  line L20 (-75.2, 52.3984) -> (-75.2, 75.2)
  line L21 (-75.2, 75.2) -> (-42.5, 75.2)
  line L22 (-42.5, 75.2) -> (-42.5, 52.3984)
  line L23 (-42.5, 52.3984) -> (-75.2, 52.3984)
  line L24 (-80, 0) -> (0, 0)
  line L25 (0, 0) -> (0, 80)
  line L26 (0, 80) -> (-80, 80)
  line L27 (-80, 80) -> (-80, 0)
  line L28 (-32.0165, 27.5498) -> (-37.5, 27.5498)
  line L29 (-37.5, 27.5498) -> (-37.5, 0)
  line L30 (-37.5, 0) -> (-32.0165, 0)
  line L31 (-32.0165, 0) -> (-32.0165, 27.5498)
  line L32 (-32.0165, 25.5269) -> (-0.0165, 25.5269) construction
  line L33 (-4.8, 27.5498) -> (-0.0165, 27.5498)
  line L34 (-0.0165, 27.5498) -> (-0.0165, 23.0269)
  line L35 (-0.0165, 23.0269) -> (-4.8, 23.0269)
  line L36 (-4.8, 23.0269) -> (-4.8, 27.5498)
  dimension "d147" = 2.5
  constraint horizontal L28
  constraint vertical L29
  constraint horizontal L30
  constraint vertical L31
  constraint coincident L24 L29.end
  constraint coincident L10.end L11.start
  constraint horizontal L33
  constraint vertical L34
  constraint horizontal L35
  constraint vertical L36
  constraint coincident L8.start L11.end
  measures "d147" distance of L32 L35
extrude "Estrusione14" add sketch "Schizzo10 (2)" along normal up to surface (3.1541 mm away) contours L8 L33 L34 L35 L36 | L10 L24 L28 L29 L30 L31 bodies 4 in component "case"
sketch "Schizzo11 (2)" plane through (-6.4703, 0, 0) normal (-1, 0, 0) x (0, -1, 0) in component "case"
  line L0 (-37.5, 0) -> (-32.0165, 0)
  line L1 (-32.0165, 0) -> (-32.0165, 27.5498)
  line L2 (-32.0165, 27.5498) -> (-37.5, 27.5498)
  line L3 (-37.5, 27.5498) -> (-37.5, 0)
  line L4 (-34.5165, 27.5498) -> (-34.5165, 0) construction
  line L5 (-34.7165, 27.5498) -> (-34.7165, 0)
  point P0 (-0.0165, 25.5269)
  point P1 (-34.5165, 23.0269)
  point P2 (-34.5165, 2.5269)
  point P3 (-32.0165, 25.5269)
  dimension "d150" = 0.2
  constraint coincident L2 L4.start
  constraint coincident L0 L4.end
  constraint perpendicular L0 L4
  constraint coincident L2 L5.start
  constraint coincident L0 L5.end
  constraint perpendicular L0 L5
  measures "d150" distance of L4 L5
extrude "Estrusione15" add sketch "Schizzo11 (2)" along normal blind 3 contours L0 L2 L3 L5 bodies 4 in component "case"
sketch "Schizzo12" plane through (0, 34.7165, 0) normal (0, -1, 0) x (1, 0, 0) in component "case"
  line L0 (-6.4703, 0) -> (-6.4703, 27.5498)
  line L1 (-6.4703, 27.5498) -> (-9.4703, 27.5498)
  line L2 (-9.4703, 27.5498) -> (-9.4703, 0)
  line L3 (-9.4703, 0) -> (-6.4703, 0)
  line L4 (-7.4703, 25.5269) -> (-7.4703, 16.8269) construction
  line L5 (-7.4703, 7.8269) -> (-7.4703, 2.0269) construction
  line L6 (-9.4703, 27.5498) -> (-7.6703, 27.5498)
  line L7 (-7.6703, 27.5498) -> (-7.6703, 21.5498)
  line L8 (-7.6703, 21.5498) -> (-9.4703, 21.5498)
  line L9 (-9.4703, 21.5498) -> (-9.4703, 27.5498)
  line L10 (-9.4703, 0) -> (-7.6703, 0)
  line L11 (-7.6703, 0) -> (-7.6703, 4)
  line L12 (-7.6703, 4) -> (-9.4703, 4)
  line L13 (-9.4703, 4) -> (-9.4703, 0)
  dimension "d153" = 6
  dimension "d154" = 0.2
  dimension "d155" = 4
  dimension "d156" = 0.2
  constraint horizontal L6
  constraint vertical L7
  constraint horizontal L8
  constraint vertical L9
  constraint coincident L1.end L2.start
  constraint horizontal L10
  constraint vertical L11
  constraint horizontal L12
  constraint vertical L13
  constraint coincident L2.end L3.start
  measures "d153" distance of L1.end L8.end
  measures "d154" distance of L4 L7
  measures "d155" distance of L2.end L12.end
  measures "d156" distance of L5 L11
extrude "Estrusione16" add sketch "Schizzo12" along normal up to surface (2.7 mm away) contours L2 L3 L10 L11 L12 L13 | L1 L2 L6 L7 L8 L9 bodies 4 in component "case"
sketch "Schizzo13" plane through (-6.4703, 0, 0) normal (-1, 0, 0) x (0, -1, 0) in component "case"
  line L0 (-4.8, 27.5498) -> (-4.8, 23.0269)
  line L1 (-4.8, 23.0269) -> (-0.0165, 23.0269)
  line L2 (-0.0165, 23.0269) -> (-0.0165, 27.5498)
  line L3 (-0.0165, 27.5498) -> (-4.8, 27.5498)
  line L4 (-4.8, 25.7269) -> (-0.0165, 25.7269)
  line L5 (-32.0165, 25.5269) -> (-0.0165, 25.5269)
  dimension "d159" = 0.2
  constraint coincident L0 L4.start
  constraint coincident L2 L4.end
  constraint perpendicular L2 L4
  measures "d159" distance of L4 L5
extrude "Estrusione17" add sketch "Schizzo13" along normal blind 3 contours L0 L2 L3 L4 bodies 4 in component "case"
sketch "Schizzo14" plane through (0, 0, 25.7269) normal (0, 0, -1) x (1, 0, 0) in component "case"
  line L0 (-6.4703, -4.8) -> (-6.4703, -0.0165)
  line L1 (-6.4703, -0.0165) -> (-9.4703, -0.0165)
  line L2 (-9.4703, -0.0165) -> (-9.4703, -4.8)
  line L3 (-9.4703, -4.8) -> (-6.4703, -4.8)
  line L4 (-9.4703, -0.0165) -> (-7.6703, -0.0165)
  line L5 (-7.6703, -0.0165) -> (-7.6703, -4.8)
  line L6 (-7.6703, -4.8) -> (-9.4703, -4.8)
  line L7 (-9.4703, -4.8) -> (-9.4703, -0.0165)
  line L8 (-7.4703, -0.0165) -> (-7.4703, -5.5165)
  dimension "d162" = 0.2
  constraint horizontal L4
  constraint vertical L5
  constraint horizontal L6
  constraint vertical L7
  constraint coincident L3 L5.end
  constraint coincident L1.end L2.start
  measures "d162" distance of L5 L8
extrude "Estrusione18" add sketch "Schizzo14" along normal up to surface (2.7 mm away) contours L1 L2 L3 L4 L5 L6 L7 bodies 4 in component "case"
sketch "Schizzo15" plane through (0, -1.8, 0) normal (0, -1, 0) x (1, 0, 0) in component "case"
  line L0 (-16, -1.8) -> (1.2, -1.8)
  line L1 (1.2, -1.8) -> (1.2, 81.8)
  line L2 (1.2, 81.8) -> (-16, 81.8)
  line L3 (-16, 81.8) -> (-16, -1.8)
  line L4 (-5.3375, 15.5269) -> (-4.5203, 15.5269)
  arc A0 (-4.4703, 15.4769) -> (-4.5203, 15.5269) centre (-4.5203, 15.4769) ccw
  line L5 (-4.4703, 15.4769) -> (-4.4703, 8.4769)
  arc A1 (-4.5203, 8.4269) -> (-4.4703, 8.4769) centre (-4.5203, 8.4769) ccw
  line L6 (-4.5203, 8.4269) -> (-5.3375, 8.4269)
  line L7 (-5.3375, 8.4269) -> (-6.2703, 9.3598)
  line L8 (-6.2703, 9.3598) -> (-6.2703, 14.5941)
  line L9 (-6.2703, 14.5941) -> (-5.3375, 15.5269)
  arc A2 (-4.5203, 8.2269) -> (-4.2703, 8.4769) centre (-4.5203, 8.4769) ccw
  line L10 (-4.2703, 8.4769) -> (-4.2703, 15.4769)
  arc A3 (-4.2703, 15.4769) -> (-4.5203, 15.7269) centre (-4.5203, 15.4769) ccw
  line L11 (-4.5203, 15.7269) -> (-5.4203, 15.7269)
  line L12 (-5.4203, 15.7269) -> (-6.4703, 14.6769)
  line L13 (-6.4703, 14.6769) -> (-6.4703, 9.2769)
  line L14 (-6.4703, 9.2769) -> (-5.4203, 8.2269)
  line L15 (-5.4203, 8.2269) -> (-4.5203, 8.2269)
  line L16 (-4.2703, -1.8) -> (-4.2703, 81.8) construction
  line L17 (1.2, 8.2269) -> (-16, 8.2269) construction
  line L18 (-4.2703, 8.2269) -> (-6.4703, 8.2269) construction
  line L19 (-6.4703, 8.2269) -> (-6.4703, 15.7269) construction
  line L20 (-6.4703, 15.7269) -> (-4.2703, 15.7269) construction
  line L21 (-4.2703, 15.7269) -> (-4.2703, 8.2269) construction
  line L22 (-6.4703, 15.7269) -> (-4.2703, 8.2269) construction
  line L23 (-6.4703, 8.2269) -> (-4.2703, 15.7269) construction
  line L24 (-9.1203, 18.2269) -> (-1.6203, 18.2269)
  line L25 (-1.6203, 18.2269) -> (-1.6203, 5.7269)
  line L26 (-1.6203, 5.7269) -> (-9.1203, 5.7269)
  line L27 (-9.1203, 5.7269) -> (-9.1203, 18.2269)
  line L28 (-9.1203, 18.2269) -> (-1.6203, 5.7269) construction
  line L29 (-1.6203, 18.2269) -> (-9.1203, 5.7269) construction
  point P0 (-5.3703, 11.9769)
  dimension "d165" = 7.5
  dimension "d166" = 12.5
  constraint coincident L0 L16.start
  constraint coincident L2 L16.end
  constraint perpendicular L2 L16
  constraint coincident L1 L17.start
  constraint coincident L3 L17.end
  constraint perpendicular L3 L17
  constraint horizontal L18
  constraint vertical L19
  constraint horizontal L20
  constraint vertical L21
  constraint coincident L17 L18.start
  constraint coincident L16 L18.start
  constraint horizontal L24
  constraint perpendicular L24 L25
  constraint parallel L24 L26
  constraint parallel L25 L27
  constraint coincident L28 P0
  constraint coincident L29 P0
  constraint midpoint L23 P0
  measures "d165" distance of L25.end L26.end
  measures "d166" distance of L24.end L25.end